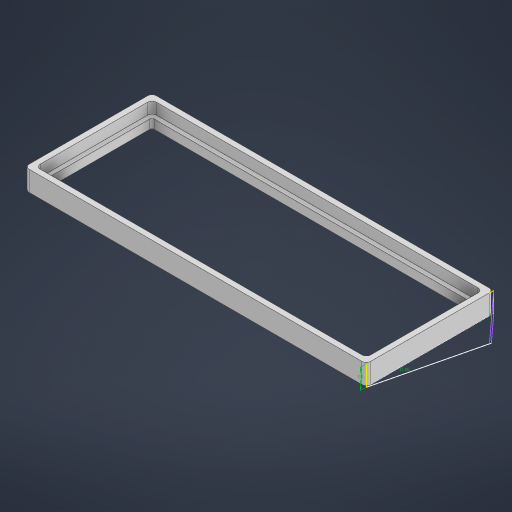
# Autodesk Inventor part: hole size and stack size
Saved by Autodesk Inventor 2024.2 (Build 282272000, 272)
## iProperties
Created: 2024-12-04
Part Number: hole size and stack size
Material: Generic
Document SubType Name: Modeling
Designer: Moe
Density: 1 g/cm^3
Appearance: Default
Author: Moe
Autodesk Inventor part; units mm, degrees
ref_plane "YZ Plane" through (0, 0, 0) normal (1, 0, 0) x (0, 1, 0)
ref_plane "XZ Plane" through (0, 0, 0) normal (0, 1, 0) x (-1, 0, 0)
ref_plane "XY Plane" through (0, 0, 0) normal (0, 0, 1) x (1, 0, 0)
sketch "Sketch1" plane through (0, 0, 0) normal (0, 1, 0) x (-1, 0, 0)
  line L0 (2, 0) -> (50, 0)
  line L1 (52, -2) -> (52, -146)
  line L2 (50, -148) -> (2, -148)
  line L3 (0, -146) -> (0, -2)
  arc A0 (52, -2) -> (50, 0) centre (50, -2) ccw
  arc A1 (0, -146) -> (2, -148) centre (2, -146) ccw
  arc A2 (50, -148) -> (52, -146) centre (50, -146) ccw
  arc A3 (2, 0) -> (0, -2) centre (2, -2) ccw
  line L4 (52.5, 2.5) -> (-0.5, 2.5)
  line L5 (-2.5, 0.5) -> (-2.5, -148.5)
  line L6 (-0.5, -150.5) -> (52.5, -150.5)
  line L7 (54.5, -148.5) -> (54.5, 0.5)
  arc A4 (54.5, 0.5) -> (52.5, 2.5) centre (52.5, 0.5) ccw
  arc A5 (-0.5, 2.5) -> (-2.5, 0.5) centre (-0.5, 0.5) ccw
  arc A6 (-2.5, -148.5) -> (-0.5, -150.5) centre (-0.5, -148.5) ccw
  arc A7 (52.5, -150.5) -> (54.5, -148.5) centre (52.5, -148.5) ccw
  point P0 (0, 0)
  point P1 (52, -148)
  point P2 (52, 0)
  point P3 (0, -148)
  dimension "d0" = 52
  dimension "d1" = 148
  dimension "d2" = 2
  dimension "d3" = 2.5
  dimension "d4" = 2.5
  dimension "d5" = 2.5
  dimension "d6" = 2.5
  dimension "d7" = 2
  constraints: 16 end point, 16 point on circle, 16 tangent, 8 centre point, 8 point on line, 6 equal radius, 4 parallel, 2 horizontal, 2 perpendicular
  measures "d0" distance of point (52, -148) point (0, -148)
  measures "d1" distance of point (52, 0) point (52, -148)
  measures "d2" radius of A0
  measures "d3" distance between parallel lines of L1 L7
  measures "d4" distance between parallel lines of L4 L0
  measures "d5" distance between parallel lines of L5 L3
  measures "d6" distance between parallel lines of L6 L2
  measures "d7" radius of A4
extrude "Extrusion1" add sketch "Sketch1" along normal blind 5
sketch "Sketch2" plane through (0, 0, 0) normal (0, -1, 0) x (1, 0, 0)
  arc A0 (2.5, 0.5) -> (0.5, 2.5) centre (0.5, 0.5) ccw projected
  line L0 (-52.5, 2.5) -> (0.5, 2.5) projected
  arc A1 (-52.5, 2.5) -> (-54.5, 0.5) centre (-52.5, 0.5) ccw projected
  line L1 (-54.5, -148.5) -> (-54.5, 0.5) projected
  arc A2 (-54.5, -148.5) -> (-52.5, -150.5) centre (-52.5, -148.5) ccw projected
  line L2 (0.5, -150.5) -> (-52.5, -150.5) projected
  arc A3 (0.5, -150.5) -> (2.5, -148.5) centre (0.5, -148.5) ccw projected
  line L3 (2.5, 0.5) -> (2.5, -148.5) projected
  line L4 (0, -146) -> (0, -2) projected
  arc A4 (-2, -148) -> (0, -146) centre (-2, -146) ccw projected
  line L5 (-50, -148) -> (-2, -148) projected
  arc A5 (-52, -146) -> (-50, -148) centre (-50, -146) ccw projected
  line L6 (-52, -2) -> (-52, -146) projected
  arc A6 (-50, 0) -> (-52, -2) centre (-50, -2) ccw projected
  line L7 (-2, 0) -> (-50, 0) projected
  arc A7 (0, -2) -> (-2, 0) centre (-2, -2) ccw projected
  line L8 (-49, -146) -> (-3, -146)
  line L9 (-2, -145) -> (-2, -3)
  line L10 (-3, -2) -> (-49, -2)
  line L11 (-50, -3) -> (-50, -145)
  arc A8 (-3, -146) -> (-2, -145) centre (-3, -145) ccw
  arc A9 (-50, -145) -> (-49, -146) centre (-49, -145) ccw
  arc A10 (-49, -2) -> (-50, -3) centre (-49, -3) ccw
  arc A11 (-2, -3) -> (-3, -2) centre (-3, -3) ccw
  point P0 (0, 0)
  dimension "d10" = 1
  constraints: 8 end point, 8 point on circle, 8 tangent, 4 centre point, 4 point on line, 3 equal radius, 2 parallel, 1 horizontal, 1 perpendicular
  measures "d10" radius of A8
extrude "Extrusion2" add sketch "Sketch2" along normal blind 2 contours L3 A3 L2 A2 L1 A1 L0 A0 | A4 L5 A5 L6 A6 L7 A7 L4
sketch "Sketch3" plane through (0, -2, 0) normal (0, -1, 0) x (1, 0, 0)
  line L0 (2.5, -148.5) -> (2.5, 0.5) projected
  arc A0 (2.5, 0.5) -> (0.5, 2.5) centre (0.5, 0.5) ccw projected
  line L1 (0.5, 2.5) -> (-52.5, 2.5) projected
  arc A1 (-52.5, 2.5) -> (-54.5, 0.5) centre (-52.5, 0.5) ccw projected
  line L2 (-54.5, 0.5) -> (-54.5, -148.5) projected
  arc A2 (-54.5, -148.5) -> (-52.5, -150.5) centre (-52.5, -148.5) ccw projected
  line L3 (-52.5, -150.5) -> (0.5, -150.5) projected
  arc A3 (0.5, -150.5) -> (2.5, -148.5) centre (0.5, -148.5) ccw projected
  arc A4 (-50, -145) -> (-49, -146) centre (-49, -145) ccw projected
  line L4 (-50, -145) -> (-50, -3) projected
  arc A5 (-49, -2) -> (-50, -3) centre (-49, -3) ccw projected
  line L5 (-49, -2) -> (-3, -2) projected
  arc A6 (-2, -3) -> (-3, -2) centre (-3, -3) ccw projected
  line L6 (-2, -3) -> (-2, -145) projected
  arc A7 (-3, -146) -> (-2, -145) centre (-3, -145) ccw projected
  line L7 (-3, -146) -> (-49, -146) projected
  point P0 (0, 0)
extrude "Extrusion3" add sketch "Sketch3" along normal blind 2
sketch "Sketch4" plane through (0.5, 5, -150.5) normal (0, 0, -1) x (-1, 0, 0)
  line L0 (-2, -9) -> (-2, 0) projected
  line L1 (-2, -9) -> (53.9521, -19.876)
  line L2 (-2, -9) -> (54.9993, -9) construction
  line L3 (55, -9) -> (55, 0) projected
  line L4 (53.9521, -19.876) -> (55, -9)
  line L5 (55, 0) -> (53, 0) projected
  line L6 (55, 0) -> (53.1086, -19.712)
  point P0 (0.5, -5)
  dimension "d15" = 11
  dimension "d16" = 9
  constraints: 8 end point, 1 equal length, 1 horizontal, 1 point on line
  measures "d15" angle of L1 L2
  measures "d16" distance of L0.start L0.end
body "Solid1"
